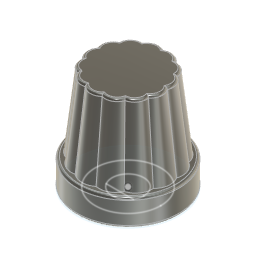
knob_normal (Autodesk Fusion 360 design; units mm, degrees)
Autodesk Fusion 360 part; units mm, degrees
sketch "Sketch1" plane through (0, 0, 0) normal (0, 0, 1) x (1, 0, 0)
  circle A0 centre (0, 0) radius 10.5
  circle A1 centre (0, 0) radius 9.5 construction
  circle A2 centre (0, 0) radius 9 construction
  line L0 (0, 0) -> (0, 9) construction
  line L1 (0, 0) -> (4.1825, 7.9691) construction
  arc A3 (4.1825, 7.9691) -> (0, 9) centre (1.4534, 5.8969) ccw
  arc A4 (0, 9) -> (-4.1825, 7.9691) centre (-1.4534, 5.8969) ccw
  arc A5 (-4.1825, 7.9691) -> (-7.4069, 5.1126) centre (-4.0274, 4.546) ccw
  arc A6 (-7.4069, 5.1126) -> (-8.9344, 1.0848) centre (-5.6787, 2.1536) ccw
  arc A7 (-8.9344, 1.0848) -> (-8.4151, -3.1914) centre (-6.0291, -0.7321) ccw
  arc A8 (-8.4151, -3.1914) -> (-5.9681, -6.7366) centre (-4.9983, -3.4501) ccw
  arc A9 (-5.9681, -6.7366) -> (-2.1538, -8.7385) centre (-2.8224, -5.3777) ccw
  arc A10 (-2.1538, -8.7385) -> (2.1538, -8.7385) centre (0, -6.0734) ccw
  arc A11 (2.1538, -8.7385) -> (5.9681, -6.7366) centre (2.8224, -5.3777) ccw
  arc A12 (5.9681, -6.7366) -> (8.4151, -3.1914) centre (4.9983, -3.4501) ccw
  arc A13 (8.4151, -3.1914) -> (8.9344, 1.0848) centre (6.0291, -0.7321) ccw
  arc A14 (8.9344, 1.0848) -> (7.4069, 5.1126) centre (5.6787, 2.1536) ccw
  arc A15 (7.4069, 5.1126) -> (4.1825, 7.9691) centre (4.0274, 4.546) ccw
  dimension "d1" = 21
  dimension "d2" = 19
  dimension "d3" = 18
  dimension "d4" = 27.692
  dimension "d6" = 360
  constraint coincident A0.centre A1.centre
  constraint concentric A0 A2
  constraint coincident A2 L0.end
  constraint vertical L0
  constraint coincident A2 L1.end
  constraint tangent A1 A3
  measures "d1" diameter of A0
  measures "d2" diameter of A1
  measures "d3" diameter of A2
  measures "d4" angle of L0 L1
ref_plane "WorkPlane1" through (0, 0, 15.5) normal (0, 0, 1) x (1, 0, 0)
sketch "Sketch2" plane through (0, 0, 15.5) normal (0, 0, 1) x (1, 0, 0)
  circle A0 centre (0, 0) radius 7.75 construction
  circle A1 centre (0, 0) radius 7.25 construction
  line L0 (0, 0) -> (0, 7.25) construction
  line L1 (0, 0) -> (3.3692, 6.4196) construction
  arc A2 (3.3692, 6.4196) -> (0, 7.25) centre (1.2628, 5.1234) ccw
  arc A3 (0, 7.25) -> (-3.3692, 6.4196) centre (-1.2628, 5.1234) ccw
  arc A4 (-3.3692, 6.4196) -> (-5.9666, 4.1185) centre (-3.4991, 3.9497) ccw
  arc A5 (-5.9666, 4.1185) -> (-7.1971, 0.8739) centre (-4.9338, 1.8711) ccw
  arc A6 (-7.1971, 0.8739) -> (-6.7789, -2.5709) centre (-5.2382, -0.636) ccw
  arc A7 (-6.7789, -2.5709) -> (-4.8076, -5.4267) centre (-4.3426, -2.9975) ccw
  arc A8 (-4.8076, -5.4267) -> (-1.735, -7.0393) centre (-2.4522, -4.6723) ccw
  arc A9 (-1.735, -7.0393) -> (1.735, -7.0393) centre (0, -5.2767) ccw
  arc A10 (1.735, -7.0393) -> (4.8076, -5.4267) centre (2.4522, -4.6723) ccw
  arc A11 (4.8076, -5.4267) -> (6.7789, -2.5709) centre (4.3426, -2.9975) ccw
  arc A12 (6.7789, -2.5709) -> (7.1971, 0.8739) centre (5.2382, -0.636) ccw
  arc A13 (7.1971, 0.8739) -> (5.9666, 4.1185) centre (4.9338, 1.8711) ccw
  arc A14 (5.9666, 4.1185) -> (3.3692, 6.4196) centre (3.4991, 3.9497) ccw
  dimension "d8" = 15.5
  dimension "d9" = 14.5
  dimension "d10" = 27.692
  dimension "d12" = 360
  constraint coincident A0.centre A1.centre
  constraint coincident A1 L0.end
  constraint vertical L0
  constraint coincident A1 L1.end
  constraint tangent A0 A2
  measures "d8" diameter of A0
  measures "d9" diameter of A1
  measures "d10" angle of L0 L1
loft "Loft1" add profiles "Sketch1", "Sketch2" section 1 contours A3 A4 A5 A6 A7 A8 A9 A10 A11 A12 A13 A14 A15 section 2
extrude "Extrude1" add sketch "Sketch1" against normal blind 5.5 contours A0 | A3 A4 A5 A6 A7 A8 A9 A10 A11 A12 A13 A14 A15
sketch "Sketch3" plane through (0, 0, -5.5) normal (0, 0, -1) x (1, 0, 0)
  circle A0 centre (0, 0) radius 10.5
  circle A1 centre (0, 0) radius 6.75
  circle A2 centre (0, 0) radius 3.25
  line L0 (-2.7699, 1.7) -> (2.7699, 1.7)
  dimension "d15" = 13.5
  dimension "d16" = 6.5
  dimension "d17" = 1.7
  constraint concentric A0 A1
  constraint concentric A1 A2
  constraint coincident A2 L0.start
  constraint coincident A2 L0.end
  constraint horizontal L0
  measures "d15" diameter of A1
  measures "d16" diameter of A2
  measures "d17" distance of A0.centre L0
extrude "Extrude2" cut sketch "Sketch3" against normal blind 19.5 contours A2 L0 picked at (-0.7022, 0.2404)
extrude "Extrude3" cut sketch "Sketch3" against normal blind 5.5 contours A1 | A2 L0 picked at (-0.7983, 2.2791)
fillet "Fillet1" radius 0.5 1 edges at (-6.2932, -2.4409, 0)
fillet "Fillet2" radius 1 1 edges at (-6.2932, -2.4409, -5.5)
fillet "Fillet3" radius 0.5 1 edges at (-9.7894, 3.797, -5.5)
fillet "Fillet4" radius 0.5 1 edges at (-9.7894, -3.797, 0)
fillet "Fillet5" radius 0.5 13 edges at (1.8547, 7.5248, 15.5) (5.1392, 5.801, 15.5) (7.2464, 2.7482, 15.5) (7.6935, -0.9342, 15.5) (6.3781, -4.4025, 15.5) (3.6016, -6.8623, 15.5) (0, -7.75, 15.5) (-3.6016, -6.8623, 15.5) (-6.3781, -4.4025, 15.5) (-7.6935, -0.9342, 15.5) (-7.2464, 2.7482, 15.5) (-5.1392, 5.801, 15.5) (-1.8547, 7.5248, 15.5)
equation "d4 = ( 360 / 13 ) * 1 deg"
equation "d10 = ( 360 / 13 ) * 1 deg"
named bodies: "knob_normal"
